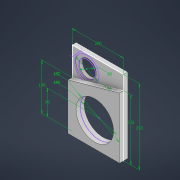
# Autodesk Inventor part: Front_L
Saved by Autodesk Inventor 2022 (Build 260153000, 153)
## iProperties
Created: 2022-04-08
Part Number: Front_L
Material: Типовые
Document SubType Name: Modeling
Designer: Kalugin_a
Density: 1 g/cm^3
Appearance: По умолчанию
Author: Kalugin_a
Autodesk Inventor part; units mm, degrees
ref_plane "YZ Plane" through (0, 0, 0) normal (1, 0, 0) x (0, 1, 0)
ref_plane "XZ Plane" through (0, 0, 0) normal (0, 1, 0) x (-1, 0, 0)
ref_plane "XY Plane" through (0, 0, 0) normal (0, 0, 1) x (1, 0, 0)
sketch "Front0" plane through (0, 0, 0) normal (0, 0, 1) x (1, 0, 0)
  line L0 (0, 0) -> (200, 0)
  line L1 (200, 0) -> (200, 290)
  line L2 (200, 290) -> (0, 290)
  line L3 (0, 290) -> (0, 0)
  circle A0 centre (104, 96) radius 73
  circle A1 centre (104, 96) radius 91
  circle A2 centre (57, 237) radius 47
  circle A3 centre (57, 237) radius 33
  line L4 (0, 180) -> (200, 236)
  line L5 (36, 290) -> (0, 250)
  line L6 (0, 87) -> (47.17, 0)
  point P0 (43.1585, 192.0844)
  point P1 (92.1531, 205.8029)
  dimension "d0" = 200
  dimension "d1" = 290
  dimension "d2" = 146
  dimension "d3" = 182
  dimension "d4" = 94
  dimension "d5" = 66
  dimension "d15" = 236
  dimension "d16" = 180
  dimension "d17" = 96
  constraints: 14 end point, 6 coincident, 6 point on line, 4 centre point, 2 parallel, 1 horizontal, 1 perpendicular
  measures "d0" distance of L2.end L1.end
  measures "d1" distance of L1.end L0.end
  measures "d2" diameter of A0
  measures "d3" diameter of A1
  measures "d4" diameter of A2
  measures "d5" diameter of A3
  measures "d15" distance of L0.end L4.end
  measures "d16" distance of L0.start L4.start
  measures "d17" distance from line of L0 A0.centre
extrude "Выдавливание2" add sketch "Front0" against normal blind 16 contours L3 L6 L0 | L6 L3 L4 A2 L1 L0 | L3 L5 L2 L1 L4 A2 | L3 L2 L5 | L4 A2 | A2 L4 | A1
extrude "Выдавливание3" cut sketch "Front0" against normal blind 4 contours L4 A2 | A2 L4 | A3
sketch "Эскиз7" plane through (0, 0, 0) normal (0, 0, 1) x (1, 0, 0)
  circle A0 centre (104, 96) radius 73
  circle A1 centre (104, 96) radius 91
  line L0 (0, 180) -> (200, 236)
  line L1 (200, 0) -> (0, 0) projected
  line L2 (0, 180) -> (0, 0)
  line L3 (200, 290) -> (200, 0) projected
  line L4 (0, 0) -> (200, 0)
  line L5 (200, 0) -> (200, 236)
  line L6 (0, 0) -> (0, 290) projected
  point P0 (43.1585, 192.0844)
  point P1 (92.1531, 205.8029)
  point P2 (47.17, 0)
  point P3 (0, 87)
  point P4 (36, 290)
  point P5 (0, 250)
  point P6 (47.17, 0)
  point P7 (0, 87)
  point P8 (35.7143, 190)
  point P9 (0, 115)
  dimension "d24" = 146
  dimension "d25" = 182
  constraints: 8 end point, 3 coincident, 2 centre point, 2 perpendicular, 2 point on line, 1 collinear
  measures "d24" diameter of A0
  measures "d25" diameter of A1
extrude "Выдавливание6" add sketch "Эскиз7" along normal blind 16 contours A1 | L0 L3 L1 L2
sketch "Эскиз8" plane through (0, 0, -16) normal (-1, 0, 0) x (0, 0, 1)
  point P0 (16, 0)
